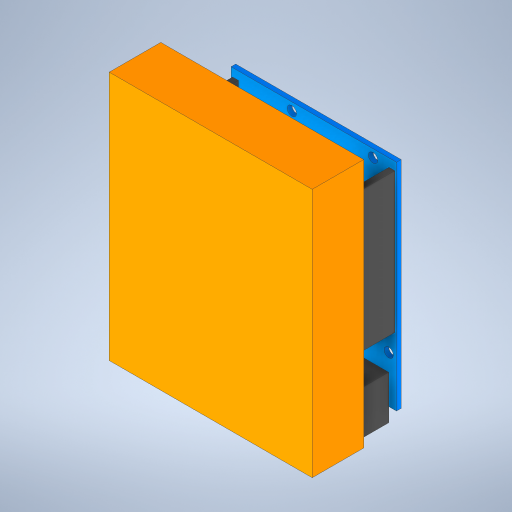
# Autodesk Inventor part: 스피커
Saved by Autodesk Inventor 2023 (Build 270158000, 158)
## iProperties
Created: 2022-11-10
Part Number: 스피커
Material: 일반
Document SubType Name: Modeling
Designer: user
Density: 1 g/cm^3
Appearance: 기본값
Author: user
Autodesk Inventor part; units mm, degrees
ref_plane "YZ Plane" through (0, 0, 0) normal (1, 0, 0) x (0, 1, 0)
ref_plane "XZ Plane" through (0, 0, 0) normal (0, 1, 0) x (-1, 0, 0)
ref_plane "XY Plane" through (0, 0, 0) normal (0, 0, 1) x (1, 0, 0)
sketch "스케치2" plane through (0, 0, 0) normal (0, 0, 1) x (1, 0, 0)
  line L0 (-26.5, -34.5) -> (26.5, -34.5)
  line L1 (26.5, -34.5) -> (26.5, 34.5)
  line L2 (26.5, 34.5) -> (-26.5, 34.5)
  line L3 (-26.5, 34.5) -> (-26.5, -34.5)
  line L4 (-26.5, -34.5) -> (26.5, 34.5) construction
  line L5 (26.5, -34.5) -> (-26.5, 34.5) construction
  circle A0 centre (19, 32) radius 1.5
  circle A1 centre (-7, 32) radius 1.5
  circle A2 centre (24, -19.5) radius 1.5
  circle A3 centre (-24, -19.5) radius 1.5
  point P0 (0, 0)
  dimension "d0" = 53
  dimension "d1" = 69
  dimension "d2" = 3
  dimension "d3" = 3
  dimension "d4" = 2.5
  dimension "d5" = 2.5
  dimension "d6" = 7.5
  dimension "d8" = 26
  dimension "d9" = 3
  dimension "d10" = 3
  dimension "d11" = 2.5
  dimension "d12" = 2.5
  dimension "d13" = 15
  constraints: 12 end point, 4 centre point, 2 midpoint, 2 parallel, 1 horizontal, 1 horizontal alignment, 1 perpendicular
  measures "d0" distance of L2.end L1.end
  measures "d1" distance of L1.end L0.end
  measures "d2" diameter of A0
  measures "d3" diameter of A1
  measures "d4" distance from line of L2 A1.centre
  measures "d5" distance from line of L2 A0.centre
  measures "d6" distance from line of L1 A0.centre
  measures "d8" distance of A0.centre A1.centre
  measures "d9" diameter of A2
  measures "d10" diameter of A3
  measures "d11" distance from line of L3 A3.centre
  measures "d12" distance from line of L1 A2.centre
  measures "d13" distance from line of L0 A2.centre
extrude "돌출1" add sketch "스케치2" along normal blind 1.5
sketch "스케치3" plane through (0, 0, 1.5) normal (0, 0, 1) x (1, 0, 0)
  line L0 (-16.5, -26.3) -> (-4.5, -26.3)
  line L1 (-4.5, -26.3) -> (-4.5, -43)
  line L2 (-4.5, -43) -> (-16.5, -43)
  line L3 (-16.5, -43) -> (-16.5, -26.3)
  line L4 (-16.5, -26.3) -> (-4.5, -43) construction
  line L5 (-4.5, -26.3) -> (-16.5, -43) construction
  line L6 (15, -25) -> (24, -25)
  line L7 (24, -25) -> (24, -39)
  line L8 (24, -39) -> (15, -39)
  line L9 (15, -39) -> (15, -25)
  line L10 (15, -25) -> (24, -39) construction
  line L11 (24, -25) -> (15, -39) construction
  line L12 (-26.5, -34.5) -> (26.5, -34.5) projected
  line L13 (26.5, -34.5) -> (26.5, 34.5) projected
  line L14 (-26.5, 34.5) -> (-26.5, -34.5) projected
  point P0 (0, 0)
  point P1 (-10.5, -34.65)
  point P2 (19.5, -32)
  dimension "d16" = 12
  dimension "d17" = 16.7
  dimension "d18" = 9
  dimension "d19" = 14
  dimension "d20" = 4.5
  dimension "d21" = 2.5
  dimension "d22" = 8.5
  dimension "d23" = 10
  constraints: 24 end point, 4 midpoint, 4 parallel, 2 horizontal, 2 perpendicular
  measures "d16" distance of L1.end L2.end
  measures "d17" distance of L0.end L1.end
  measures "d18" distance of L7.end L8.end
  measures "d19" distance of L6.end L7.end
  measures "d20" distance between parallel lines of L12 L8
  measures "d21" distance between parallel lines of L13 L7
  measures "d22" distance between parallel lines of L12 L2
  measures "d23" distance between parallel lines of L14 L3
extrude "돌출2" add sketch "스케치3" along normal blind 11 contours L0 L1 L12 L3 | L12 L1 L2 L3
extrude "돌출3" add sketch "스케치3" along normal blind 11 contours L6 L7 L12 L9 | L12 L7 L8 L9
sketch "스케치4" plane through (0, 0, 1.5) normal (0, 0, 1) x (1, 0, 0)
  line L0 (-25.9905, -12.9426) -> (-24.0965, -12.9426)
  line L1 (-24.0965, -12.9426) -> (-24.0965, 31.8831)
  line L2 (-24.0965, 31.8831) -> (-25.9905, 31.8831)
  line L3 (-25.9905, 31.8831) -> (-25.9905, -12.9426)
  line L4 (-25.9905, -12.9426) -> (-24.0965, 31.8831) construction
  line L5 (-24.0965, -12.9426) -> (-25.9905, 31.8831) construction
  line L6 (0, 0) -> (0, 9.4702)
  line L7 (25.9905, -12.9426) -> (24.0965, -12.9426)
  line L8 (24.0965, -12.9426) -> (24.0965, 31.8831)
  line L9 (24.0965, 31.8831) -> (25.9905, 31.8831)
  line L10 (25.9905, 31.8831) -> (25.9905, -12.9426)
  line L11 (25.9905, -12.9426) -> (24.0965, 31.8831) construction
  line L12 (24.0965, -12.9426) -> (25.9905, 31.8831) construction
  point P0 (-25.0435, 9.4702)
  point P1 (25.0435, 9.4702)
  constraints: 26 end point, 5 symmetric about line, 2 midpoint, 2 parallel, 1 horizontal, 1 perpendicular, 1 vertical
extrude "돌출4" add sketch "스케치4" along normal blind 11
sketch "스케치5" plane through (0, 0, 12.5) normal (0, 0, 1) x (1, 0, 0)
  line L0 (-38, -39) -> (27, -39)
  line L1 (27, -39) -> (27, 41)
  line L2 (27, 41) -> (-38, 41)
  line L3 (-38, 41) -> (-38, -39)
  line L4 (-38, -39) -> (27, 41) construction
  line L5 (27, -39) -> (-38, 41) construction
  line L6 (26.5, -34.5) -> (26.5, 34.5) projected
  point P0 (0, 0)
  point P1 (-5.5, 1)
  point P2 (-38, 34.5)
  point P3 (24, -39)
  dimension "d30" = 80
  dimension "d31" = 65
  dimension "d34" = 0.5
  constraints: 12 end point, 2 midpoint, 2 parallel, 2 point on line, 1 horizontal, 1 perpendicular
  measures "d30" distance of L0.end L1.end
  measures "d31" distance of L1.end L2.end
  measures "d34" distance between parallel lines of L1 L6
extrude "돌출5" add sketch "스케치5" along normal blind 16.5
